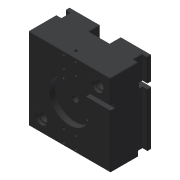
# Autodesk Inventor part: topplate1
Saved by Autodesk Inventor 2022 Beta2 (Build 260130000, 130) ContinuousBuild 0
## iProperties
Shininess: 64.0
Length Units: 11272
Angle Units: 11279
Time Units: 11290
Mass Units: 11286
Length Display Precision: 3
Angle Display Precision: 2
Compacted: True
Part Number: topplate1
Document SubType Name: Modeling
Created: 2003-04-03
Designer: Sudhir John
Density: 1 g/cm^3
Material: Generic
Appearance: Generic
Density: 0.0
Volumn: 0.0
Area: 0.0
PropertySet Name: Model Information
Control State: 0
Master: False
Checked Out: False
Author: Sudhir John
Autodesk Inventor part; units mm, degrees
ref_plane "YZ Plane" through (0, 0, 0) normal (1, 0, 0) x (0, 1, 0)
sketch "Sketch1" plane through (0, 0, 0) normal (0, 0, 1) x (1, 0, 0)
  line L0 (-19.2506, -177.8124) -> (183.9494, -177.8124)
  line L1 (183.9494, -177.8124) -> (183.9494, 25.3876)
  line L2 (183.9494, 25.3876) -> (-19.2506, 25.3876)
  line L3 (-19.2506, 25.3876) -> (-19.2506, -177.8124)
  dimension "d0" = 203.2
  constraints: 8 end point, 2 parallel, 1 horizontal, 1 perpendicular
  measures "d0" distance of L1.end L2.end
extrude "Extrusion1" add sketch "Sketch1" along normal blind 101.6
sketch "Sketch2" plane through (-19.2506, -177.8124, 0) normal (0, -1, 0) x (1, 0, 0)
  line L0 (0, 0) -> (0, 101.6) projected
  line L1 (203.2, 0) -> (203.2, 101.6) projected
  line L2 (0, 10.16) -> (12.368, 10.16)
  line L3 (12.368, 10.16) -> (12.368, 32.385)
  line L4 (12.368, 32.385) -> (0, 32.385)
  dimension "d4" = 10.16
  dimension "d5" = 22.225
  constraints: 6 end point, 2 perpendicular, 2 point on line, 1 parallel
  measures "d4" distance of L2.start L0.start
  measures "d5" distance of L4.end L2.start
extrude "side cut left" cut sketch "Sketch2" against normal through all
ref_plane "Work Plane1" through (82.3494, -177.8124, 0) normal (1, 0, 0) x (0, 0, -1)
mirror "side cut mirror" about plane through (82.3494, -177.8124, 0) normal (1, 0, 0) of "side cut left"
sketch "Sketch3" plane through (0, 0, 101.6) normal (0, 0, 1) x (1, 0, 0)
  line L0 (-19.2506, -177.8124) -> (-19.2506, 25.3876) projected
  line L1 (183.9494, -177.8124) -> (-19.2506, -177.8124) projected
  line L2 (183.9494, 25.3876) -> (183.9494, -177.8124) projected
  line L3 (-19.2506, 25.3876) -> (183.9494, 25.3876) projected
  line L4 (12.4994, -6.3624) -> (12.4994, -146.0624)
  line L5 (12.4994, -146.0624) -> (152.1994, -146.0624)
  line L6 (152.1994, -146.0624) -> (152.1994, -6.3624)
  line L7 (152.1994, -6.3624) -> (12.4994, -6.3624)
  dimension "d8" = 31.75
  constraints: 8 end point, 2 coincident, 3 other
  measures "d8" distance between parallel lines of L0 L4
hole "Pin c'bore Hole1" at (12.4994, -146.0624, 101.6) at (152.1994, -6.3624, 101.6) direction (0, 0, -1) diameter 22.2377 end through all counterbore diameter 29.21 counterbore depth 6.604
sketch "Sketch4" plane through (0, 0, 101.6) normal (0, 0, 1) x (1, 0, 0)
  circle A0 centre (82.3494, -76.2124) radius 8.001
  dimension "d16" = 16.002
  constraints: 1 centre point
  measures "d16" diameter of A0
extrude "center bore" cut sketch "Sketch4" against normal through all
sketch "Sketch5" plane through (0, 0, 101.6) normal (0, 0, 1) x (1, 0, 0)
  circle A0 centre (82.3494, -76.2124) radius 8.001 projected
  circle A1 centre (82.3494, -76.2124) radius 50.1904
  dimension "d19" = 100.3808
  constraints: 1 centre point, 1 coincident, 1 concentric
  measures "d19" diameter of A1
extrude "Top counterbore" cut sketch "Sketch5" against normal blind 13.97
sketch "Sketch6" plane through (0, 0, 0) normal (0, 0, -1) x (-1, 0, 0)
  circle A0 centre (-82.3494, -76.2124) radius 8.001 projected
  circle A1 centre (-82.3494, -76.2124) radius 8.3312
  dimension "d22" = 16.6624
  constraints: 1 centre point, 1 coincident, 1 concentric
  measures "d22" diameter of A1
extrude "Extrusion5" cut sketch "Sketch6" against normal blind 24.0332 contours A0 | A1
sketch "Sketch8" plane through (0, 0, 0) normal (0, 0, -1) x (-1, 0, 0)
  circle A0 centre (-82.3494, -76.2124) radius 8.3312 projected
  circle A1 centre (-82.3494, -76.2124) radius 18.161
  dimension "d25" = 36.322
  constraints: 1 centre point, 1 coincident, 1 concentric
  measures "d25" diameter of A1
extrude "C'bore bottom" cut sketch "Sketch8" against normal blind 11.2898
ref_plane "Work Plane2" through (-19.2506, -76.2124, 0) normal (0, 1, 0) x (1, 0, 0)
sketch "Sketch9" plane through (0, 0, 0) normal (0, 0, -1) x (-1, 0, 0)
  line L0 (19.2506, -177.8124) -> (-183.9494, -177.8124) projected
  line L1 (-183.9494, -177.8124) -> (-183.9494, 25.3876) projected
  line L2 (-244.9094, -76.2124) -> (39.5706, -76.2124) projected
  line L3 (-82.3494, -198.1324) -> (-82.3494, 86.3476) projected
  circle A0 centre (-82.3494, -76.2124) radius 50.1904 projected
  circle A1 centre (-82.3494, -76.2124) radius 42.8625 construction
  point P0 (-125.2119, -161.9374)
  point P1 (-39.4869, -161.9374)
  point P2 (-125.2119, 9.5126)
  point P3 (-39.4869, 9.5126)
  point P4 (-125.2119, -76.2124)
  point P5 (-39.4869, -76.2124)
  point P6 (-82.3494, -119.0749)
  point P7 (-82.3494, -33.3499)
  dimension "d28" = 15.875
  dimension "d29" = 58.7375
  constraints: 4 point on line, 3 point on circle, 3 symmetric about line, 1 centre point, 1 coincident
  measures "d28" distance from line of L0 point (-125.212, -161.937)
  measures "d29" distance from line of L1 point (-125.212, -161.937)
hole "Hole2" at (125.2119, -161.9374, 0) at (39.4869, -161.9374, 0) at (125.2119, 9.5126, 0) at (39.4869, 9.5126, 0) at (125.2119, -76.2124, 0) at (39.4869, -76.2124, 0) at (82.3494, -119.0749, 0) at (82.3494, -33.3499, 0) direction (0, 0, 1) diameter 6.4008 depth 20.32 tip angle 118 thread size "5/16-18 UNC" class "1B" standard "ANSI Unified Screw Threads"
sketch "Sketch10" plane through (82.3494, -76.2124, 87.63) normal (0, 0, 1) x (1, 0, 0)
  circle A0 centre (0, 0) radius 50.1904 projected
  circle A1 centre (0, 0) radius 42.0624
  line L0 (0, 0) -> (-32.3289, 32.3289)
  line L1 (0, 0) -> (32.3289, -32.3289)
  point P0 (-29.7426, 29.7426)
  point P1 (29.7426, -29.7426)
  dimension "d37" = 84.1248
  constraints: 4 end point, 2 point on circle, 2 point on line, 1 centre point, 1 collinear, 1 concentric
  measures "d37" diameter of A1
hole "Hole3" at (52.6067, -46.4698, 87.63) at (112.092, -105.955, 87.63) direction (0, 0, -1) diameter 6.4008 depth 22.1361 tip angle 118 thread size "5/16-18 UNC" class "1B" standard "ANSI Unified Screw Threads"
chamfer "Chamfer1" distance 0.3175 distance2 0.1842 1 edges at (74.3484, -76.2124, 24.0332) measured on face at (89.8662, -73.0178, 24.0332)
sketch "Sketch11" plane through (82.3494, -76.2124, 11.2898) normal (0, 0, -1) x (-1, 0, 0)
  circle A0 centre (0, 0) radius 18.161 projected
  line L0 (0, 0) -> (-15.3979, 8.89)
  line L1 (0, 0) -> (15.3979, -8.89)
  circle A1 centre (0, 0) radius 12.192
  point P0 (-10.5586, 6.096)
  point P1 (10.5586, -6.096)
  dimension "d47" = 24.384
  constraints: 4 end point, 2 point on circle, 2 point on line, 1 centre point, 1 coincident, 1 collinear, 1 concentric
  measures "d47" diameter of A1
hole "Hole4" at (92.9079, -70.1164, 11.2898) at (71.7908, -82.3084, 11.2898) direction (0, 0, 1) diameter 6.4008 depth 13.589 tip angle 118 thread size "5/16-18 UNC" class "1B" standard "ANSI Unified Screw Threads"
sketch "Sketch12" plane through (-19.2506, -177.8124, 0) normal (0, -1, 0) x (1, 0, 0)
  line L0 (0, 0) -> (203.2, 0) projected
  line L1 (101.6, 132.08) -> (101.6, -10.16) projected
  line L2 (76.2, 0) -> (76.2, 27.686)
  line L3 (76.2, 27.686) -> (127, 27.686)
  line L4 (127, 27.686) -> (127, 0)
  dimension "d55" = 50.8
  dimension "d56" = 25.4
  dimension "d57" = 27.686
  constraints: 6 end point, 2 parallel, 2 point on line, 1 perpendicular
  measures "d55" distance of L4.end L2.start
  measures "d56" distance from line of L1 L4.end
  measures "d57" distance of L3.end L4.end
extrude "Extrusion7" cut sketch "Sketch12" against normal blind 45.72
mirror "Mirror3" about plane through (-19.2506, -76.2124, 0) normal (0, 1, 0) of "Extrusion7"
sketch "Sketch13" plane through (-19.2506, -177.8124, 101.6) normal (0, -1, 0) x (1, 0, 0)
  line L0 (203.2, 0) -> (0, 0) projected
  line L1 (101.6, 30.48) -> (101.6, -111.76) projected
  point P0 (101.6, -15.875)
  dimension "d60" = 15.875
  constraints: 1 point on line
  measures "d60" distance from line of L0 point (101.6, -15.875)
hole "Hole5" at (82.3494, -177.8124, 85.725) direction (0, 1, 0) diameter 6.4008 depth 32.4612 tip angle 118 thread size "5/16-18 UNC" class "1B" standard "ANSI Unified Screw Threads"
mirror "Mirror2" about plane through (-19.2506, -76.2124, 0) normal (0, 1, 0) of "Hole5"
sketch "Sketch14" plane through (107.7494, -177.8124, 27.686) normal (0, 0, -1) x (-1, 0, 0)
  line L0 (50.8, 0) -> (0, 0) projected
  line L1 (25.4, -20.32) -> (25.4, 264.16) projected
  point P0 (10.414, 7.112)
  point P1 (40.386, 7.112)
  point P2 (10.414, 37.084)
  point P3 (40.386, 37.084)
  dimension "d69" = 14.986
  dimension "d70" = 7.112
  dimension "d71" = 29.972
  constraints: 1 symmetric about line
  measures "d69" distance from line of L1 point (10.414, 7.112)
  measures "d70" distance from line of L0 point (10.414, 7.112)
  measures "d71" distance of point (10.414, 37.084) point (10.414, 7.112)
hole "Hole6" at (97.3354, -170.7004, 27.686) at (67.3634, -170.7004, 27.686) at (97.3354, -140.7284, 27.686) at (67.3634, -140.7284, 27.686) direction (0, 0, 1) diameter 6.4008 end through all thread size "5/16-18 UNC" class "1B" standard "ANSI Unified Screw Threads"
mirror "Mirror4" about plane through (-19.2506, -76.2124, 0) normal (0, 1, 0) of "Hole6"
sketch "Sketch17" plane through (0, 0, 101.6) normal (0, 0, 1) x (1, 0, 0)
  circle A0 centre (82.3494, -76.2124) radius 50.1904 projected
  line L0 (183.9494, 25.3876) -> (183.9494, -177.8124) projected
  line L1 (-19.2506, 25.3876) -> (183.9494, 25.3876) projected
  line L2 (183.9494, -31.7624) -> (122.0275, -31.7624)
  line L3 (183.9494, -44.4624) -> (124.1317, -44.4624)
  line L4 (122.0443, -45.4977) -> (122.3357, -45.2064)
  line L5 (113.064, -36.5175) -> (114.8433, -34.7382)
  arc A1 (122.0275, -31.7624) -> (114.8433, -34.7382) centre (122.0275, -41.9224) ccw
  arc A2 (124.1317, -44.4624) -> (122.3357, -45.2064) centre (124.1317, -47.0024) ccw
  line L6 (82.3494, -76.2124) -> (88.0069, -70.5548)
  line L7 (126.7994, -31.7624) -> (127.2506, -31.3111)
  circle A3 centre (82.3494, -76.2124) radius 8.001 projected
  dimension "d82" = 57.15
  dimension "d83" = 12.7
  dimension "d85" = 12.7
  dimension "d86" = 10.16
  dimension "d87" = 2.54
  constraints: 12 end point, 6 point on circle, 4 tangent, 3 point on line, 2 centre point, 2 parallel, 2 other
  measures "d82" distance between parallel lines of L1 L2
  measures "d83" distance between parallel lines of L3 L2
  measures "d85" distance between parallel lines of L5 L4
  measures "d86" radius of A1
  measures "d87" radius of A2
extrude "Extrusion8" cut sketch "Sketch17" against normal blind 10.922 contours A0 L5 A1 L2 L0 L3 A2 L4
sketch "Sketch18" plane through (0, 0, 0) normal (0, 0, -1) x (-1, 0, 0)
  circle A0 centre (-82.3494, -76.2124) radius 18.161 projected
  line L0 (-183.9494, -177.8124) -> (-183.9494, 25.3876) projected
  line L1 (-183.9494, -31.7624) -> (-122.0275, -31.7624) projected
  line L2 (-124.1317, -44.4624) -> (-183.9494, -44.4624) projected
  arc A1 (-114.8433, -34.7382) -> (-122.0275, -31.7624) centre (-122.0275, -41.9224) ccw projected
  line L3 (-114.8433, -34.7382) -> (-113.064, -36.5175) projected
  arc A2 (-122.3357, -45.2064) -> (-124.1317, -44.4624) centre (-124.1317, -47.0024) ccw projected
  line L4 (-122.0443, -45.4977) -> (-122.3357, -45.2064) projected
  line L5 (-89.8904, -59.6911) -> (-114.8433, -34.7382)
  line L6 (-98.8707, -68.6713) -> (-122.0443, -45.4977)
  constraints: 4 end point, 2 point on circle, 1 parallel, 1 tangent
extrude "Extrusion9" cut sketch "Sketch18" against normal blind 18.8214 contours A0 L6 L4 A2 L2 L0 L1 A1 L3 L5
chamfer "Chamfer2" distance 1.27 angle 45 17 edges at (-19.2506, -76.2124, 101.6) (82.3494, 25.3876, 101.6) (183.9494, -3.1874, 101.6) (183.9494, -111.1374, 101.6) (82.3494, -177.8124, 101.6) (183.9494, -76.2124, 32.385) (183.9494, -111.1374, 10.16) (183.9494, -3.1874, 10.16) (183.9494, -3.1874, 0) (183.9494, -111.1374, 0) (145.8494, 25.3876, 0) (18.8494, 25.3876, 0) (-19.2506, -76.2124, 0) (-19.2506, -76.2124, 10.16) (-19.2506, -76.2124, 32.385) (145.8494, -177.8124, 0) (18.8494, -177.8124, 0)
chamfer "Chamfer3" distance 1.27 angle 45 20 edges at (183.9494, 25.3876, 5.08) (183.9494, 25.3876, 66.9925) (177.1303, 25.3876, 32.385) (171.5813, 25.3876, 21.2725) (177.1303, 25.3876, 10.16) (-19.2506, 25.3876, 5.08) (-19.2506, 25.3876, 66.9925) (-12.4316, 25.3876, 32.385) (-6.8826, 25.3876, 21.2725) (-12.4316, 25.3876, 10.16) (183.9494, -177.8124, 5.08) (183.9494, -177.8124, 66.9925) (177.1303, -177.8124, 32.385) (171.5813, -177.8124, 21.2725) (177.1303, -177.8124, 10.16) (-19.2506, -177.8124, 5.08) (-19.2506, -177.8124, 66.9925) (-12.4316, -177.8124, 32.385) (-6.8826, -177.8124, 21.2725) (-12.4316, -177.8124, 10.16)
chamfer "Chamfer4" distance 1.27 angle 45 12 edges at (56.9494, 25.3876, 14.478) (56.9494, 1.8926, 0) (82.3494, -20.3324, 0) (107.7494, 1.8926, 0) (107.7494, 25.3876, 14.478) (82.3494, 25.3876, 27.686) (82.3494, -132.0924, 0) (56.9494, -154.3174, 0) (107.7494, -154.3174, 0) (107.7494, -177.8124, 14.478) (82.3494, -177.8124, 27.686) (56.9494, -177.8124, 14.478)
body "Solid1"
